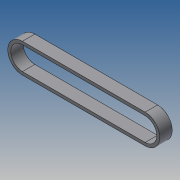
# Autodesk Inventor part: BBP MCMASTER 1679K116_BELT
Saved by Autodesk Inventor 2018.3 (Build 223284000, 284)
## iProperties
Created: 2019-09-11
Part Number: BBP MCMASTER 1679K116_BELT
Material: Generic
Vendor: HHMI: JRC - ID&F
Document SubType Name: Modeling
Designer: arnoldj
Density: 1 g/cm^3
Appearance: Default
RuleStatus: InUse
AfterDocSave0: file://Part Number Cleaner
Author: arnoldj
Revision Number: 0
DESIGN DEPARTMENT: HHMI: JRC - ID&F
ALTERED ITEM PART NUMBER: N/A
ALTERED ITEM VENDOR: N/A
ALTERED ITEM DESCRIPTION: N/A
Autodesk Inventor part; units mm, degrees
ref_plane "YZ Plane" through (0, 0, 0) normal (1, 0, 0) x (0, 1, 0)
ref_plane "XZ Plane" through (0, 0, 0) normal (0, 1, 0) x (-1, 0, 0)
ref_plane "XY Plane" through (0, 0, 0) normal (0, 0, 1) x (1, 0, 0)
sketch "Sketch1" plane through (0, 0, 0) normal (0, 0, 1) x (1, 0, 0)
  line L0 (0, 15.666) -> (0, -15.666) projected
  line L1 (-34.4366, 0) -> (128.2896, 0) projected
  line L2 (0, 0) -> (93.853, 0) construction
  line L3 (0, 8.89) -> (93.853, 8.89)
  line L4 (0, -8.89) -> (93.853, -8.89)
  arc A0 (0, 8.89) -> (0, -8.89) centre (0, 0) ccw
  arc A1 (93.853, -8.89) -> (93.853, 8.89) centre (93.853, 0) ccw
  line L5 (93.853, 11.19) -> (0, 11.19)
  arc A2 (0, 11.19) -> (0, -11.19) centre (0, 0) ccw
  line L6 (0, -11.19) -> (93.853, -11.19)
  arc A3 (93.853, -11.19) -> (93.853, 11.19) centre (93.853, 0) ccw
  dimension "d0" = 93.853
  dimension "d5" = 8.89
  dimension "d6" = 8.89
  dimension "d7" = 2.3
  constraints: 10 end point, 8 point on circle, 4 centre point, 4 tangent, 2 coincident, 1 point on line, 3 other
  measures "d0" distance of L2.start L2.end
  measures "d5" radius of A0
  measures "d6" radius of A1
  measures "d7" distance between parallel lines of L3 L5
extrude "Extrusion1" add sketch "Sketch1" along normal blind 9.525 contours L5 A3 L1 A1 L3 L0 | L0 A0 L1 A2 | L1 A0 L0 A2 | A3 L6 L0 L4 A1 L1
body "Solid1"
